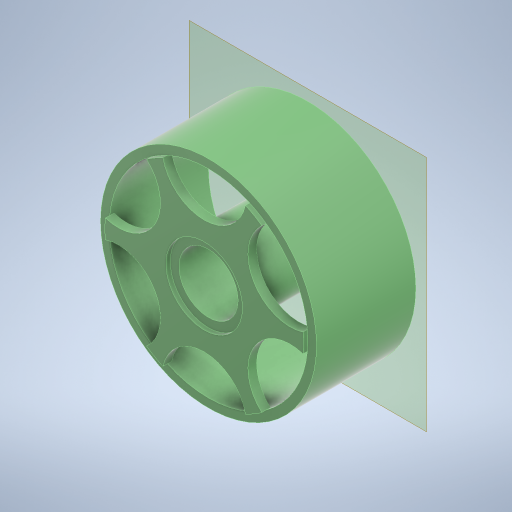
# Autodesk Inventor part: wheel
Saved by Autodesk Inventor 2023 (Build 270158000, 158)
## iProperties
Created: 2023-09-13
Part Number: wheel
Material: Iron, Cast
Document SubType Name: Modeling
Designer: 1908174
Density: 7.15 g/cm^3
Appearance: Smooth - Dark Forest Green
Author: 1908174
Autodesk Inventor part; units mm, degrees
ref_plane "YZ Plane" through (0, 0, 0) normal (1, 0, 0) x (0, 1, 0)
ref_plane "XZ Plane" through (0, 0, 0) normal (0, 1, 0) x (-1, 0, 0)
ref_plane "XY Plane" through (0, 0, 0) normal (0, 0, 1) x (1, 0, 0)
sketch "Sketch1" plane through (0, 0, 0) normal (0, 0, 1) x (1, 0, 0)
  circle A0 centre (0, 0) radius 5.588
  circle A1 centre (0, 0) radius 4.318
  circle A2 centre (0, 0) radius 14.478
  circle A3 centre (0, 0) radius 15.748
  dimension "d0" = 11.176
  dimension "d1" = 1.27
  dimension "d2" = 8.89
  dimension "d3" = 1.27
  constraints: 4 centre point, 1 coincident
  measures "d0" diameter of A0
  measures "d1" radial gap between concentric circles of A0 A1
  measures "d2" radial gap between concentric circles of A0 A2
  measures "d3" radial gap between concentric circles of A2 A3
extrude "Extrusion1" add sketch "Sketch1" along normal blind 14.478
ref_plane "Work Plane1" through (0, 0, 0) normal (0, 0, -1) x (-1, 0, 0)
sketch "Sketch2" plane through (0, 0, 14.478) normal (0, 0, 1) x (1, 0, 0)
  circle A0 centre (0, 0) radius 15.748 projected
  circle A1 centre (0, 0) radius 14.478 projected
  circle A2 centre (0, 0) radius 5.588 projected
  circle A3 centre (0, 0) radius 4.318 projected
extrude "Extrusion2" add sketch "Sketch2" along normal mid plane 1.27 contours A1
sketch "Sketch3" plane through (0, 0, 15.113) normal (0, 0, 1) x (1, 0, 0)
  circle A0 centre (0, 0) radius 14.478 projected
  arc A1 (-6.0209, 13.1667) -> (6.0209, 13.1667) centre (0, 14.478) ccw
  arc A2 (-14.4131, 1.3691) -> (-8.3923, 11.7976) centre (-12.5383, 7.239) ccw
  arc A3 (-8.3923, -11.7976) -> (-14.4131, -1.3691) centre (-12.5383, -7.239) ccw
  arc A4 (6.0209, -13.1667) -> (-6.0209, -13.1667) centre (0, -14.478) ccw
  arc A5 (14.4131, -1.3691) -> (8.3923, -11.7976) centre (12.5383, -7.239) ccw
  arc A6 (8.3923, 11.7976) -> (14.4131, 1.3691) centre (12.5383, 7.239) ccw
  point P0 (14.4131, 1.3691)
  point P1 (-8.3923, 11.7976)
  point P2 (-14.4131, 1.3691)
  point P3 (-14.4131, -1.3691)
  point P4 (-8.3923, -11.7976)
  point P5 (6.0209, -13.1667)
  point P6 (14.4131, -1.3691)
  dimension "d11" = 360
  constraints: 15 point on circle, 6 centre point, 25 other
extrude "Extrusion4" cut sketch "Sketch3" against normal blind 1.27 contours A6 A0 | A0 A5 | A1 A0 | A0 A4 | A2 A0 | A0 A3
body "Solid1"
